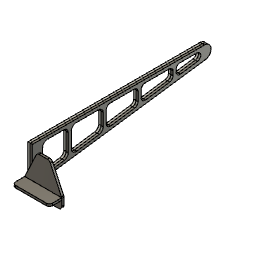
arm v3 (Autodesk Fusion 360 design; units mm, degrees)
Autodesk Fusion 360 part; units mm, degrees
note: some values were not read from the file. Chosen so that the rebuilt part matches the saved one: which face or edge a step refers to. Set by a fixed rule: which sketch regions a step uses.
sketch "Sketch1" plane through (0, 0, 0) normal (0, 0, 1) x (1, 0, 0)
  line L0 (0, 0) -> (304.8, 0)
  line L1 (304.8, 0) -> (304.8, 304.8)
  line L2 (304.8, 304.8) -> (0, 304.8)
  line L3 (0, 304.8) -> (0, 0)
  line L4 (152.4, 0) -> (152.4, 79.629) construction
  line L5 (228.6, 70.358) -> (76.2, 70.358)
  line L6 (76.2, 70.358) -> (76.2, 88.9)
  line L7 (76.2, 88.9) -> (228.6, 88.9)
  line L8 (228.6, 88.9) -> (228.6, 70.358)
  line L9 (228.6, 70.358) -> (76.2, 88.9) construction
  line L10 (76.2, 70.358) -> (228.6, 88.9) construction
  line L11 (0, 0) -> (0, 88.9) construction
  line L12 (304.8, 0) -> (304.8, 88.9) construction
  line L13 (152.4, 304.8) -> (203.2, 304.8) construction
  line L14 (152.4, 304.8) -> (101.6, 304.8) construction
  line L15 (0, 88.9) -> (101.6, 304.8)
  line L16 (203.2, 304.8) -> (304.8, 88.9)
  point P0 (152.4, 79.629)
  dimension "d1" = 304.8
  dimension "d2" = 304.8
  dimension "d3" = 79.629
  dimension "d4" = 152.4
  dimension "d5" = 18.542
  dimension "d6" = 88.9
  dimension "d7" = 88.9
  dimension "d8" = 50.8
  dimension "d9" = 50.8
  constraint horizontal L0
  constraint vertical L1
  constraint horizontal L2
  constraint vertical L3
  constraint coincident L0.start L3.end
  constraint midpoint L0 L4.start
  constraint perpendicular L0 L4
  constraint horizontal L5
  constraint perpendicular L5 L6
  constraint parallel L5 L7
  constraint parallel L6 L8
  constraint coincident L9 P0
  constraint coincident L10 P0
  constraint coincident P0 L4.end
  constraint perpendicular L0 L11
  constraint perpendicular L0 L12
  constraint midpoint L2 L13.start
  constraint parallel L2 L13
  constraint parallel L2 L14
  measures "d1" distance of L0.start L0.end
  measures "d2" distance of L0.start L2.end
  measures "d3" distance of L4.start P0
  measures "d4" distance of L6.end L7.end
  measures "d5" distance of L5.end L6.end
  measures "d6" distance of L0.start L11.end
  measures "d7" distance of L0.end L12.end
  measures "d8" distance of L13.start L13.end
  measures "d9" distance of L13.start L14.end
extrude "Extrude1" add sketch "Sketch1" along normal blind 18.288 contours L0 L1 L2 L3 L15 L16 makes body 1 in component "Component"
fillet "Fillet1" radius 25.4 6 edges at (203.2, 304.8, 9.144) (101.6, 304.8, 9.144) (304.8, 88.9, 9.144) (304.8, 0, 9.144) (0, 88.9, 9.144) (0, 0, 9.144) on bodies 1 in component "Component"
sketch "Sketch2" plane through (0, 0, 0) normal (0, 0, -1) x (-1, 0, 0)
  line L0 (-228.6, 88.9) -> (-76.2, 88.9)
  line L1 (-76.2, 88.9) -> (-76.2, 70.358)
  line L2 (-76.2, 70.358) -> (-228.6, 70.358)
  line L3 (-228.6, 70.358) -> (-228.6, 88.9)
  arc A0 (-25.4, 0) -> (0, 25.4) centre (-25.4, 25.4) ccw
  line L4 (0, 25.4) -> (0, 83.2222)
  arc A1 (0, 83.2222) -> (-2.4176, 94.0374) centre (-25.4, 83.2222) ccw
  line L5 (-2.4176, 94.0374) -> (-94.7366, 290.2152)
  arc A2 (-94.7366, 290.2152) -> (-117.719, 304.8) centre (-117.719, 279.4) ccw
  line L6 (-117.719, 304.8) -> (-187.081, 304.8)
  arc A3 (-187.081, 304.8) -> (-210.0634, 290.2152) centre (-187.081, 279.4) ccw
  line L7 (-210.0634, 290.2152) -> (-302.3824, 94.0374)
  arc A4 (-302.3824, 94.0374) -> (-304.8, 83.2222) centre (-279.4, 83.2222) ccw
  line L8 (-304.8, 83.2222) -> (-304.8, 25.4)
  arc A5 (-304.8, 25.4) -> (-279.4, 0) centre (-279.4, 25.4) ccw
  line L9 (-279.4, 0) -> (-25.4, 0)
  line L10 (-152.4, 88.9) -> (-152.4, 79.629) construction
  line L11 (0, 70.358) -> (-304.8, 70.358)
  line L12 (-304.8, 70.358) -> (-304.8, 88.9)
  line L13 (-304.8, 88.9) -> (0, 88.9)
  line L14 (0, 88.9) -> (0, 70.358)
  line L15 (0, 70.358) -> (-304.8, 88.9) construction
  line L16 (-304.8, 70.358) -> (0, 88.9) construction
  point P0 (-152.4, 79.629)
  dimension "d14" = 9.271
  constraint midpoint L0 L10.start
  constraint perpendicular L2 L10
  constraint horizontal L11
  constraint perpendicular L11 L12
  constraint parallel L11 L13
  constraint parallel L12 L14
  constraint coincident L4 L11.start
  constraint coincident L15 P0
  constraint coincident L16 P0
  constraint coincident P0 L10.end
  measures "d14" distance of L10.start P0
extrude "Extrude1'" add sketch "Sketch2" against normal blind 101.6 separate body contours L0 L1 L2 L3 L11 L13 | L3 A4 L8 L11 L12 L13 | L1 L4 A1 L11 L13 L14 | A4 L12 L13 | A1 L13 L14 makes body 2 in component "Component'"
extrude "Extrude2" add sketch "Sketch2" along normal blind 18.542 contours L0 L1 L2 L3 L11 L13 bodies 2 in component "Component'"
fillet "Fillet1'" radius 25.4 2 edges at (0, 79.629, 101.6) (304.8, 79.629, 101.6) on bodies 2 in component "Component'"
sketch "Sketch3" plane through (0, 0, 0) normal (1, 0, 0) x (0, 0, -1)
  line L0 (0, 0) -> (25.4, 0) construction
  line L1 (25.4, 0) -> (25.4, 304.8)
  line L2 (25.4, 304.8) -> (1498.6, 304.8)
  line L3 (1498.6, 304.8) -> (1498.6, 203.2)
  line L4 (1498.6, 203.2) -> (25.4, 0)
  line L5 (25.4, 304.8) -> (279.4, 304.8) construction
  line L6 (1498.6, 304.8) -> (1498.6, 279.4) construction
  line L7 (1498.6, 203.2) -> (1498.6, 228.6) construction
  line L8 (1498.6, 228.6) -> (1473.2, 228.6) construction
  line L9 (1498.6, 279.4) -> (1473.2, 279.4) construction
  line L10 (25.4, 304.8) -> (25.4, 279.4) construction
  line L11 (25.4, 279.4) -> (50.8, 279.4) construction
  line L12 (25.4, 0) -> (25.4, 25.4) construction
  line L13 (25.4, 25.4) -> (50.8, 25.4) construction
  line L14 (1473.2, 279.4) -> (50.8, 279.4)
  line L15 (50.8, 279.4) -> (50.8, 25.4)
  line L16 (50.8, 25.4) -> (1473.2, 228.6)
  line L17 (1473.2, 228.6) -> (1473.2, 279.4)
  line L18 (1473.2, 279.4) -> (1210.7333, 279.4) construction
  line L19 (1210.7333, 279.4) -> (1185.3333, 279.4) construction
  line L20 (1185.3333, 279.4) -> (922.8667, 279.4) construction
  line L21 (922.8667, 279.4) -> (897.4667, 279.4) construction
  line L22 (897.4667, 279.4) -> (635, 279.4) construction
  line L23 (635, 279.4) -> (609.6, 279.4) construction
  line L24 (609.6, 279.4) -> (347.1333, 279.4) construction
  line L25 (347.1333, 279.4) -> (321.7333, 279.4) construction
  line L26 (321.7333, 279.4) -> (59.2667, 279.4) construction
  line L27 (59.2667, 279.4) -> (33.8667, 279.4) construction
  line L28 (33.8667, 279.4) -> (-228.6, 279.4) construction
  line L29 (-228.6, 279.4) -> (-228.6, -14.5143)
  line L30 (33.8667, 279.4) -> (33.8667, 22.981)
  line L31 (59.2667, 279.4) -> (59.2667, 26.6095)
  line L32 (321.7333, 279.4) -> (321.7333, 64.1048)
  line L33 (347.1333, 279.4) -> (347.1333, 67.7333)
  line L34 (609.6, 279.4) -> (609.6, 105.2286)
  line L35 (635, 279.4) -> (635, 108.8571)
  line L36 (897.4667, 279.4) -> (897.4667, 146.3524)
  line L37 (922.8667, 279.4) -> (922.8667, 149.981)
  line L38 (1185.3333, 279.4) -> (1185.3333, 187.4762)
  line L39 (1210.7333, 279.4) -> (1210.7333, 191.1048)
  dimension "d21" = 25.4
  dimension "d22" = 304.8
  dimension "d23" = 1473.2
  dimension "d24" = 101.6
  dimension "d25" = 25.4
  dimension "d26" = 25.4
  dimension "d27" = 25.4
  dimension "d28" = 25.4
  dimension "d29" = 25.4
  dimension "d30" = 25.4
  dimension "d31" = 25.4
  dimension "d32" = 25.4
  dimension "d33" = 262.4667
  dimension "d34" = 25.4
  dimension "d35" = 262.4667
  dimension "d36" = 25.4
  dimension "d37" = 262.4667
  dimension "d38" = 25.4
  dimension "d39" = 262.4667
  dimension "d40" = 25.4
  dimension "d41" = 262.4667
  dimension "d42" = 25.4
  dimension "d43" = 262.4667
  constraint coincident L0.start origin
  constraint horizontal L0
  constraint perpendicular L0 L1
  constraint perpendicular L1 L2
  constraint perpendicular L2 L3
  constraint coincident L2 L5.end
  constraint vertical L6
  constraint vertical L7
  constraint perpendicular L7 L8
  constraint perpendicular L3 L9
  constraint perpendicular L2 L10
  constraint perpendicular L10 L11
  constraint perpendicular L0 L12
  constraint perpendicular L1 L13
  constraint perpendicular L1 L18
  constraint parallel L14 L19
  constraint parallel L14 L20
  constraint parallel L14 L21
  constraint parallel L14 L22
  constraint parallel L14 L23
  constraint parallel L14 L24
  constraint parallel L14 L25
  constraint parallel L14 L26
  constraint parallel L14 L27
  constraint perpendicular L15 L28
  constraint coincident L16 L29.end
  constraint perpendicular L14 L29
  constraint coincident L16 L30.end
  constraint perpendicular L27 L30
  constraint coincident L16 L31.end
  constraint perpendicular L14 L31
  constraint coincident L16 L32.end
  constraint perpendicular L25 L32
  constraint coincident L16 L33.end
  constraint perpendicular L14 L33
  constraint coincident L16 L34.end
  constraint perpendicular L23 L34
  constraint coincident L16 L35.end
  constraint perpendicular L14 L35
  constraint coincident L16 L36.end
  constraint perpendicular L22 L36
  constraint coincident L16 L37.end
  constraint perpendicular L21 L37
  constraint coincident L16 L38.end
  constraint perpendicular L14 L38
  constraint coincident L16 L39.end
  constraint perpendicular L18 L39
  measures "d21" distance of L0.start L0.end
  measures "d22" distance of L0.end L1.end
  measures "d23" distance of L1.end L2.end
  measures "d24" distance of L2.end L3.end
  measures "d25" distance of L2.end L6.end
  measures "d26" distance of L3.end L7.end
  measures "d27" distance of L7.end L8.end
  measures "d28" distance of L6.end L9.end
  measures "d29" distance of L1.end L10.end
  measures "d30" distance of L10.end L11.end
  measures "d31" distance of L0.end L12.end
  measures "d32" distance of L12.end L13.end
  measures "d33" distance of L9.end L18.end
  measures "d34" distance of L18.end L19.end
  measures "d35" distance of L19.end L20.end
  measures "d36" distance of L20.end L21.end
  measures "d37" distance of L21.end L22.end
  measures "d38" distance of L22.end L23.end
  measures "d39" distance of L23.end L24.end
  measures "d40" distance of L24.end L25.end
  measures "d41" distance of L25.end L26.end
  measures "d42" distance of L26.end L27.end
  measures "d43" distance of L27.end L28.end
extrude "Extrude1''" add sketch "Sketch3" along normal blind 18.542 separate body contours L1 L2 L3 L4 | L14 L16 L38 L39 | L14 L16 L36 L37 | L14 L16 L34 L35 | L14 L16 L32 L33 | L14 L15 L16 L31 makes body 3 in component "Component''"
fillet "Fillet1''" radius 38.1 8 edges at (9.271, 279.4, -609.6) (9.271, 279.4, -347.1333) (9.271, 105.2286, -609.6) (9.271, 67.7333, -347.1333) (9.271, 279.4, -321.7333) (9.271, 279.4, -59.2667) (9.271, 64.1048, -321.7333) (9.271, 26.6095, -59.2667) on bodies 3 in component "Component''"
fillet "Fillet2" radius 31.75 12 edges at (9.271, 279.4, -897.4667) (9.271, 279.4, -635) (9.271, 108.8571, -635) (9.271, 146.3524, -897.4667) (9.271, 187.4762, -1185.3333) (9.271, 149.981, -922.8667) (9.271, 279.4, -922.8667) (9.271, 279.4, -1185.3333) (9.271, 279.4, -1473.2) (9.271, 228.6, -1473.2) (9.271, 279.4, -1210.7333) (9.271, 191.1048, -1210.7333) on bodies 3 in component "Component''"
fillet "Fillet3" radius 53.848 2 edges at (9.271, 304.8, -1498.6) (9.271, 203.2, -1498.6) on bodies 3 in component "Component''"
sketch "Sketch4" plane through (0, 0, 0) normal (-1, 0, 0) x (0, 0, 1)
  arc A0 (-959.1068, 155.1581) -> (-922.8667, 186.589) centre (-954.6167, 186.589) ccw
  line L0 (-959.1068, 155.1581) -> (-1158.0735, 183.5819)
  arc A1 (-1185.3333, 215.0128) -> (-1158.0735, 183.5819) centre (-1153.5833, 215.0128) ccw
  line L1 (-1185.3333, 215.0128) -> (-1185.3333, 247.65)
  arc A2 (-1153.5833, 279.4) -> (-1185.3333, 247.65) centre (-1153.5833, 247.65) ccw
  line L2 (-1153.5833, 279.4) -> (-954.6167, 279.4)
  arc A3 (-922.8667, 247.65) -> (-954.6167, 279.4) centre (-954.6167, 247.65) ccw
  line L3 (-922.8667, 247.65) -> (-922.8667, 186.589)
  arc A4 (-1382.0436, 279.4) -> (-1386.5337, 216.2191) centre (-1382.0436, 247.65) ccw
  line L4 (-1382.0436, 279.4) -> (-1242.4833, 279.4)
  arc A5 (-1210.7333, 247.65) -> (-1242.4833, 279.4) centre (-1242.4833, 247.65) ccw
  line L5 (-1210.7333, 247.65) -> (-1210.7333, 227.7128)
  arc A6 (-1246.9735, 196.2819) -> (-1210.7333, 227.7128) centre (-1242.4833, 227.7128) ccw
  line L6 (-1246.9735, 196.2819) -> (-1386.5337, 216.2191)
  arc A7 (-671.2401, 114.0343) -> (-635, 145.4652) centre (-666.75, 145.4652) ccw
  line L7 (-671.2401, 114.0343) -> (-870.2068, 142.4581)
  arc A8 (-897.4667, 173.889) -> (-870.2068, 142.4581) centre (-865.7167, 173.889) ccw
  line L8 (-897.4667, 173.889) -> (-897.4667, 247.65)
  arc A9 (-865.7167, 279.4) -> (-897.4667, 247.65) centre (-865.7167, 247.65) ccw
  line L9 (-865.7167, 279.4) -> (-666.75, 279.4)
  arc A10 (-635, 247.65) -> (-666.75, 279.4) centre (-666.75, 247.65) ccw
  line L10 (-635, 247.65) -> (-635, 145.4652)
  arc A11 (-390.6215, 73.9459) -> (-347.1333, 111.663) centre (-385.2333, 111.663) ccw
  line L11 (-390.6215, 73.9459) -> (-576.8882, 100.5554)
  arc A12 (-609.6, 138.2725) -> (-576.8882, 100.5554) centre (-571.5, 138.2725) ccw
  line L12 (-609.6, 138.2725) -> (-609.6, 241.3)
  arc A13 (-571.5, 279.4) -> (-609.6, 241.3) centre (-571.5, 241.3) ccw
  line L13 (-571.5, 279.4) -> (-385.2333, 279.4)
  arc A14 (-347.1333, 241.3) -> (-385.2333, 279.4) centre (-385.2333, 241.3) ccw
  line L14 (-347.1333, 241.3) -> (-347.1333, 111.663)
  arc A15 (-102.7548, 32.8221) -> (-59.2667, 70.5392) centre (-97.3667, 70.5392) ccw
  line L15 (-102.7548, 32.8221) -> (-289.0215, 59.4316)
  arc A16 (-321.7333, 97.1487) -> (-289.0215, 59.4316) centre (-283.6333, 97.1487) ccw
  line L16 (-321.7333, 97.1487) -> (-321.7333, 241.3)
  arc A17 (-283.6333, 279.4) -> (-321.7333, 241.3) centre (-283.6333, 241.3) ccw
  line L17 (-283.6333, 279.4) -> (-97.3667, 279.4)
  arc A18 (-59.2667, 241.3) -> (-97.3667, 279.4) centre (-97.3667, 241.3) ccw
  line L18 (-59.2667, 241.3) -> (-59.2667, 70.5392)
  arc A19 (-1498.6, 250.1305) -> (-1452.1097, 196.7875) centre (-1444.752, 250.1305) ccw
  line L19 (-1452.1097, 196.7875) -> (-25.4, 0)
  line L20 (-25.4, 0) -> (-25.4, 304.8)
  line L21 (-25.4, 304.8) -> (-1444.752, 304.8)
  arc A20 (-1444.752, 304.8) -> (-1498.6, 250.952) centre (-1444.752, 250.952) ccw
  line L22 (-1498.6, 250.952) -> (-1498.6, 250.1305)
extrude "Extrude1'''" add sketch "Sketch4" along normal blind 18.542 separate body makes body 4 in component "Component'''"
move_face "OffsetFaces1" offset 50.8 1 faces at (6.1807, 184.3797, -59.2667) on bodies 3 in component "Component''"
move_face "OffsetFaces1'" offset 50.8 1 faces at (-6.1807, 184.3797, -59.2667) on bodies 4 in component "Component'''"
ref_plane "WorkPlane1" through (76.2, 70.358, 0) normal (0, 0, 1) x (1, 0, 0)
sketch "Sketch6" plane through (76.2, 70.358, 0) normal (0, 0, 1) x (1, 0, 0)
  line L0 (152.4, 0) -> (0, 0) construction
  line L1 (0, 0) -> (0, 18.542) construction
  line L2 (0, 0) -> (2.2451, 2.2451) construction
  circle A0 centre (2.2451, 2.2451) radius 3.175
  dimension "d79" = 3.175
  constraint coincident L0.end L1.start
  constraint coincident L0.end A0
  measures "d79" distance of L0.end L2.end
sweep "Sweep1" cut kept parallel profiles "Sketch6" along 1 edges at (76.2, 70.358, 9.144) section 1 on bodies 1 bodies 1 in component "Component"
ref_plane "WorkPlane2" through (228.6, 70.358, 0) normal (0, 0, 1) x (1, 0, 0)
sketch "Sketch7" plane through (228.6, 70.358, 0) normal (0, 0, 1) x (1, 0, 0)
  line L0 (0, 18.542) -> (0, 0) construction
  line L1 (0, 0) -> (-147.9099, 0) construction
  line L2 (0, 0) -> (-2.2451, 2.2451) construction
  circle A0 centre (-2.2451, 2.2451) radius 3.175
  dimension "d87" = 3.175
  constraint coincident L0.end L1.start
  constraint coincident L0.end A0
  measures "d87" distance of L0.end L2.end
sweep "Sweep2" cut kept parallel profiles "Sketch7" along 1 edges at (228.6, 70.358, 9.144) section 1 on bodies 1 bodies 1 in component "Component"
ref_plane "WorkPlane3" through (228.6, 88.9, 0) normal (0, 0, 1) x (1, 0, 0)
sketch "Sketch8" plane through (228.6, 88.9, 0) normal (0, 0, 1) x (1, 0, 0)
  line L0 (-152.4, 0) -> (0, 0) construction
  line L1 (0, 0) -> (0, -14.0519) construction
  line L2 (0, 0) -> (-2.2451, -2.2451) construction
  circle A0 centre (-2.2451, -2.2451) radius 3.175
  dimension "d95" = 3.175
  constraint coincident L0.end L1.start
  constraint coincident L0.end A0
  measures "d95" distance of L0.end L2.end
sweep "Sweep3" cut kept parallel profiles "Sketch8" along 1 edges at (228.6, 88.9, 9.144) section 1 on bodies 1 bodies 1 in component "Component"
ref_plane "WorkPlane4" through (76.2, 88.9, 0) normal (0, 0, 1) x (1, 0, 0)
sketch "Sketch9" plane through (76.2, 88.9, 0) normal (0, 0, 1) x (1, 0, 0)
  line L0 (0, 0) -> (147.9099, 0) construction
  line L1 (0, -14.0519) -> (0, 0) construction
  line L2 (0, 0) -> (2.2451, -2.2451) construction
  circle A0 centre (2.2451, -2.2451) radius 3.175
  dimension "d103" = 3.175
  constraint coincident L0.start L1.end
  constraint coincident L0.start A0
  measures "d103" distance of L0.start L2.end
sweep "Sweep4" cut kept parallel profiles "Sketch9" along 1 edges at (76.2, 88.9, 9.144) section 1 on bodies 1 bodies 1 in component "Component"
ref_plane "WorkPlane5" through (76.2, 88.9, 18.542) normal (0, -1, 0) x (1, 0, 0)
sketch "Sketch10" plane through (76.2, 88.9, 18.542) normal (0, -1, 0) x (1, 0, 0)
  line L0 (-76.2, 0) -> (0, 0) construction
  line L1 (0, 0) -> (0, -18.542) construction
  line L2 (0, 0) -> (-2.2451, -2.2451) construction
  circle A0 centre (-2.2451, -2.2451) radius 3.175
  dimension "d111" = 3.175
  constraint coincident L0.end L1.start
  constraint coincident L0.end A0
  measures "d111" distance of L0.end L2.end
sweep "Sweep1'" cut kept parallel profiles "Sketch10" along 1 edges at (76.2, 79.629, 0) section 1 sketch seen with x (1, 0, 0) y (0, 1, 0) z (0, 0, 1) at (0, 0, -18.542) on bodies 2 bodies 2 in component "Component'"
ref_plane "WorkPlane6" through (228.6, 70.358, 18.542) normal (0, 1, 0) x (-1, 0, 0)
sketch "Sketch11" plane through (228.6, 70.358, 18.542) normal (0, 1, 0) x (-1, 0, 0)
  line L0 (-76.2, 0) -> (0, 0) construction
  line L1 (0, 0) -> (0, -18.542) construction
  line L2 (0, 0) -> (-2.2451, -2.2451) construction
  circle A0 centre (-2.2451, -2.2451) radius 3.175
  dimension "d119" = 3.175
  constraint coincident L0.end L1.start
  constraint coincident L0.end A0
  measures "d119" distance of L0.end L2.end
sweep "Sweep2'" cut kept parallel profiles "Sketch11" along 1 edges at (228.6, 79.629, 0) section 1 sketch seen with x (1, 0, 0) y (0, 1, 0) z (0, 0, 1) at (0, 0, -18.542) on bodies 2 bodies 2 in component "Component'"
component "Component" placed x (1, 0, 0) y (0, 1, 0) z (0, 0, 1) at (0, 0, 0)
component "Component'" placed x (1, 0, 0) y (0, 1, 0) z (0, 0, 1) at (0, 0, 18.542)
component "Component''" placed x (1, 0, 0) y (0, 1, 0) z (0, 0, 1) at (0, 0, 0)
component "Component'''" placed x (1, 0, 0) y (0, 1, 0) z (0, 0, 1) at (0, 0, 0)
equation "d3 = 3.5 in - ( 0.73 / 2 ) * 1 in"
equation "d14 = ( 0.730 / 2 ) * 1 in"
equation "d33 = ( 62 / 6 ) * 1 in"
equation "d35 = ( 62 / 6 ) * 1 in"
equation "d37 = ( 62 / 6 ) * 1 in"
equation "d39 = ( 62 / 6 ) * 1 in"
equation "d41 = ( 62 / 6 ) * 1 in"
equation "d43 = ( 62 / 6 ) * 1 in"
equation "d79 = 0.25 in / 2 + 0.00 in"
equation "d87 = 0.25 in / 2 + 0.00 in"
equation "d95 = 0.25 in / 2 + 0.00 in"
equation "d103 = 0.25 in / 2 + 0.00 in"
equation "d111 = 0.25 in / 2 + 0.00 in"
equation "d119 = 0.25 in / 2 + 0.00 in"
